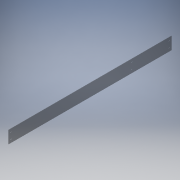
# Autodesk Inventor part: Bumper Support Plate
Saved by Autodesk Inventor 2019.4 (Build 234330000, 330)
## iProperties
Created: 2019-12-14
Part Number: Bumper Support Plate
Material: Polycarbonate, Smoke
Document SubType Name: Modeling
Designer: admin
Density: 1.2 g/cm^3
Appearance: Polycarbonate - Smoked
Author: admin
Autodesk Inventor part; units mm, degrees
ref_plane "YZ Plane" through (0, 0, 0) normal (1, 0, 0) x (0, 1, 0)
ref_plane "XZ Plane" through (0, 0, 0) normal (0, 1, 0) x (-1, 0, 0)
ref_plane "XY Plane" through (0, 0, 0) normal (0, 0, 1) x (1, 0, 0)
sketch "Sketch1" plane through (0, 0, 0) normal (1, 0, 0) x (0, 1, 0)
  line L0 (0, 0) -> (60, 0)
  line L1 (60, 0) -> (60, -800)
  line L2 (60, -800) -> (0, -800)
  line L3 (0, -800) -> (0, 0)
  dimension "d0" = 800
  dimension "d1" = 60
  constraints: 8 end point, 2 parallel, 1 horizontal, 1 perpendicular
  measures "d0" distance of L0.end L1.end
  measures "d1" distance of L0.start L0.end
extrude "Extrusion1" add sketch "Sketch1" along normal blind 2
sketch "Sketch2" plane through (2, 0, 0) normal (1, 0, 0) x (0, 0, -1)
  circle A0 centre (12.5, 45) radius 2.75
  circle A1 centre (12.5, 15) radius 2.75
  line L0 (0, 0) -> (800, 0) projected
  line L1 (0, 60) -> (0, 0) projected
  circle A2 centre (787.5, 45) radius 2.75
  line L2 (800, 0) -> (800, 60) projected
  circle A3 centre (787.5, 15) radius 2.75
  line L3 (800, 60) -> (0, 60) projected
  circle A4 centre (605, 45) radius 2.75
  circle A5 centre (605, 15) radius 2.75
  circle A6 centre (185, 45) radius 2.75
  circle A7 centre (185, 15) radius 2.75
  circle A8 centre (325, 45) radius 2.75
  circle A9 centre (325, 15) radius 2.75
  dimension "d4" = 5.5
  dimension "d5" = 5.5
  dimension "d6" = 30
  dimension "d7" = 15
  dimension "d8" = 12.5
  dimension "d9" = 12.5
  dimension "d10" = 5.5
  dimension "d11" = 12.5
  dimension "d12" = 5.5
  dimension "d13" = 12.5
  dimension "d14" = 15
  dimension "d16" = 15
  dimension "d17" = 5.5
  dimension "d18" = 5.5
  dimension "d19" = 15
  dimension "d20" = 15
  dimension "d21" = 195
  dimension "d22" = 195
  dimension "d25" = 5.5
  dimension "d26" = 5.5
  dimension "d27" = 30
  dimension "d28" = 15
  dimension "d29" = 185
  dimension "d30" = 185
  dimension "d31" = 5.5
  dimension "d32" = 5.5
  dimension "d33" = 15
  dimension "d34" = 15
  dimension "d35" = 325
  dimension "d36" = 325
  constraints: 10 centre point
  measures "d4" diameter of A0
  measures "d5" diameter of A1
  measures "d6" distance of A0.centre A1.centre
  measures "d7" distance from line of L0 A1.centre
  measures "d8" distance from line of L1 A1.centre
  measures "d9" distance from line of L1 A0.centre
  measures "d10" diameter of A2
  measures "d11" distance from line of L2 A2.centre
  measures "d12" diameter of A3
  measures "d13" distance from line of L2 A3.centre
  measures "d14" distance from line of L0 A3.centre
  measures "d16" distance from line of L3 A2.centre
  measures "d17" diameter of A4
  measures "d18" diameter of A5
  measures "d19" distance from line of L0 A5.centre
  measures "d20" distance from line of L3 A4.centre
  measures "d21" distance from line of L2 A4.centre
  measures "d22" distance from line of L2 A5.centre
  measures "d25" diameter of A6
  measures "d26" diameter of A7
  measures "d27" distance of A6.centre A7.centre
  measures "d28" distance from line of L0 A7.centre
  measures "d29" distance from line of L1 A6.centre
  measures "d30" distance from line of L1 A7.centre
  measures "d31" diameter of A8
  measures "d32" diameter of A9
  measures "d33" distance from line of L0 A9.centre
  measures "d34" distance from line of L3 A8.centre
  measures "d35" distance from line of L1 A8.centre
  measures "d36" distance from line of L1 A9.centre
extrude "Extrusion2" cut sketch "Sketch2" against normal blind 10 contours A0 | A1 | A2 | A3 | A4 | A5 | A6 | A7 | A8 | A9
body "Solid1"
